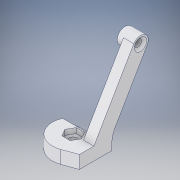
# Autodesk Inventor part: Wheelholder
Saved by Autodesk Inventor 2019.4 (Build 234330000, 330)
## iProperties
Created: 2019-04-21
Part Number: Wheelholder
Material: Пластик АБС
Document SubType Name: Modeling
Designer: NoName
Density: 1.06 g/cm^3
Appearance: PTFE
Author: NoName
Autodesk Inventor part; units mm, degrees
ref_plane "YZ Plane" through (0, 0, 0) normal (1, 0, 0) x (0, 1, 0)
ref_plane "XZ Plane" through (0, 0, 0) normal (0, 1, 0) x (-1, 0, 0)
sketch "Эскиз1" plane through (0, 0, 0) normal (0, 1, 0) x (-1, 0, 0)
  circle A0 centre (0, 0) radius 1.4
  arc A1 (5.5622, -5.7499) -> (-8, 0) centre (0, 0) ccw
  line L0 (5.5622, -5.7499) -> (-4, -15)
  line L1 (-4, -15) -> (-8, -15)
  line L2 (-8, -15) -> (-8, 0)
  line L3 (-8, 0) -> (-8, 5.6017)
  line L4 (-8, 5.6017) -> (-2.7362, 7.5175)
  line L5 (-2.7362, 7.5175) -> (-8, 0)
  point P0 (-6, -15)
  dimension "d0" = 2.8
  dimension "d1" = 8
  dimension "d3" = 15
  dimension "d4" = 4
  dimension "d46" = 110
  constraints: 12 end point, 3 point on circle, 3 tangent, 2 centre point, 2 coincident, 1 horizontal, 1 horizontal alignment, 1 midpoint, 1 vertical, 1 vertical alignment
  measures "d0" diameter of A0
  measures "d1" radius of A1
  measures "d3" distance from line of L1 point (0, 0)
  measures "d4" distance of L0.end L1.end
  measures "d46" angle of L4 L3
extrude "Выдавливание1" add sketch "Эскиз1" along normal blind 5 contours A0 | L0 L1 L2 L5 A1 | L5 A1 | A1 L3 L4
sketch "Эскиз2" plane through (0, 5, 0) normal (0, 1, 0) x (1, 0, 0)
  line L0 (-3.1754, 0) -> (-1.5877, 2.75)
  line L1 (-1.5877, 2.75) -> (1.5877, 2.75)
  line L2 (1.5877, 2.75) -> (3.1754, 0)
  line L3 (3.1754, 0) -> (1.5877, -2.75)
  line L4 (1.5877, -2.75) -> (-1.5877, -2.75)
  line L5 (-1.5877, -2.75) -> (-3.1754, 0)
  point P0 (0, 0)
  point P1 (0, 0)
  dimension "d8" = 5.5
  constraints: 12 end point, 1 coincident, 13 other
  measures "d8" distance between parallel lines of L1 L4
extrude "Выдавливание2" cut sketch "Эскиз2" against normal blind 2
ref_plane "РабПлоскость1" through (-4, 0, 0) normal (1, 0, 0) x (0, 0, -1)
sketch "Эскиз5" plane through (8, 0, 0) normal (1, 0, 0) x (0, 0, -1)
  line L0 (5.7499, 5) -> (-8, 5) projected
  circle A0 centre (18, 30) radius 1.4
  arc A1 (20.5937, 28.4925) -> (15.4063, 31.5075) centre (18, 30) ccw
  line L1 (0, 5) -> (15.4063, 31.5075)
  line L2 (15, 0) -> (15, 5) projected
  line L3 (-5.6017, 5) -> (15, 5) projected
  line L4 (0, 5) -> (0, 3) projected
  line L5 (0, 5) -> (-8, 5)
  line L6 (-8, 0) -> (-8, 5) projected
  line L7 (-8, 0) -> (-8, 5) projected
  line L8 (5.7499, 0) -> (5.7499, 5) projected
  line L9 (-8, 0) -> (5.7499, 0)
  line L10 (6.9398, 5) -> (20.5937, 28.4925)
  line L11 (5.7499, 0) -> (6.9398, 5)
  point P0 (0, 0)
  dimension "d24" = 2.8
  dimension "d38" = 25
  dimension "d40" = 3
  dimension "d45" = 3
  constraints: 10 end point, 2 centre point, 2 perpendicular, 2 point on circle, 2 point on line, 2 tangent, 1 coincident, 1 parallel
  measures "d24" diameter of A0
  measures "d38" distance from line of L3 A0.centre
  measures "d40" radius of A1
  measures "d45" distance from line of L2 A0.centre
extrude "Выдавливание4" add sketch "Эскиз5" against normal blind 4 contours L0 L1 A1 L10 L3
sketch "Эскиз6" plane through (4, 0, 0) normal (-1, 0, 0) x (0, 0, 1)
  circle A0 centre (-18, 30) radius 1.4 projected
  line L0 (-15, 0) -> (-15, 5) projected
  line L1 (-15, 0) -> (-13, 0)
  arc A1 (-13, 0) -> (-3.2532, 5) centre (-13, 12) ccw
  line L2 (-3.2532, 5) -> (-15, 5)
  line L3 (-15, 0) -> (-15, 28.4925) projected
  line L4 (-15, 0) -> (-15, 5)
  point P0 (0, 0)
  point P1 (-20.5937, 28.4925)
  point P2 (0, 5)
  dimension "d27" = 12
  constraints: 6 end point, 2 horizontal, 2 point on circle, 1 centre point, 1 collinear, 1 horizontal alignment, 1 point on line, 1 tangent, 2 other
  measures "d27" radius of A1
extrude "Выдавливание5" cut sketch "Эскиз6" along normal up to next contours L0 L2 A1 L1
chamfer "Фаска1" distance 1 angle 45 1 edges at (8, 30, -16.6)
sketch "Эскиз7" plane through (4, 0, 0) normal (-1, 0, 0) x (0, 0, 1)
  arc A0 (-15.4063, 31.5075) -> (-20.5937, 28.4925) centre (-18, 30) ccw projected
  circle A1 centre (-18, 30) radius 3
  circle A2 centre (-18, 30) radius 1.4
  point P0 (0, 0)
  dimension "d33" = 2.8
  constraints: 2 coincident, 1 centre point, 4 other
  measures "d33" diameter of A2
extrude "Выдавливание6" add sketch "Эскиз7" along normal blind 2
sketch "Эскиз10" plane through (8, 0, 0) normal (1, 0, 0) x (0, 0, -1)
  line L0 (6.9398, 5) -> (20.5937, 28.4925) projected
  line L1 (6.9398, 5) -> (6.9398, 0)
  line L2 (0, 0) -> (15, 0) projected
  line L3 (6.9398, 5) -> (15, 5) projected
  line L4 (6.9398, 5) -> (15, 5)
  line L5 (15, 5) -> (15, 0)
  constraints: 6 end point, 1 collinear, 1 perpendicular, 1 point on line, 1 vertical
extrude "Выдавливание7" cut sketch "Эскиз10" against normal up to next
sketch "Эскиз11" plane through (2, 30, -18) normal (-1, 0, 0) x (0, 0, 1)
  point P0 (18, -30)
fillet "Сопряжение1" radius 9 1 edges at (6, 5, -6.9398)
sketch "Эскиз12" plane through (0, 3, 0) normal (0, 1, 0) x (1, 0, 0)
  point P0 (0, 0)
  point P1 (0, 0)
  constraints: 1 coincident
hole "Отверстие1" at (0, 3, 0) direction (0, -1, 0) diameter 3 end through all
